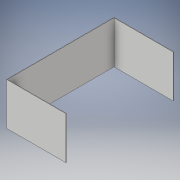
# Autodesk Inventor part: IntakeBackPlate
Saved by Autodesk Inventor 2017 (Build 210142000, 142)
## iProperties
Created: 2020-02-20
Part Number: IntakeBackPlate
Material: Generic
Document SubType Name: Modeling
Designer: S338674153
Density: 1 g/cm^3
Appearance: Default
Author: S338674153
Autodesk Inventor part; units mm, degrees
ref_plane "YZ Plane" through (0, 0, 0) normal (1, 0, 0) x (0, 1, 0)
ref_plane "XZ Plane" through (0, 0, 0) normal (0, 1, 0) x (-1, 0, 0)
ref_plane "XY Plane" through (0, 0, 0) normal (0, 0, 1) x (1, 0, 0)
sketch "Sketch1" plane through (0, 0, 0) normal (0, 1, 0) x (-1, 0, 0)
  line L0 (0, 0) -> (231.775, 0)
  line L1 (231.775, 0) -> (231.775, -4.1774)
  line L2 (229.87, -1.905) -> (0, -1.905)
  line L3 (0, -1.905) -> (0, 0)
  line L4 (231.775, 0) -> (9.6932, 0)
  line L5 (229.87, -1.905) -> (229.87, -417.195)
  line L6 (9.6932, -419.1) -> (231.775, -419.1)
  line L7 (231.775, -419.1) -> (231.775, 0)
  line L8 (231.775, -419.1) -> (0, -419.1)
  line L9 (0, -419.1) -> (0, -417.195)
  line L10 (0, -417.195) -> (229.87, -417.195)
  line L11 (231.775, -13.6272) -> (231.775, -419.1)
  dimension "d0" = 419.1
  dimension "d1" = 231.775
  dimension "d2" = 1.905
  dimension "d3" = 1.905
  dimension "d4" = 1.905
  constraints: 24 end point, 6 parallel, 3 horizontal, 3 perpendicular, 1 point on line
  measures "d0" distance of L6.end L0.end
  measures "d1" distance of L6.end L8.end
  measures "d2" distance of L8.end L9.end
  measures "d3" distance of L2.end L0.start
  measures "d4" distance between parallel lines of L7 L5
extrude "Extrusion1" add sketch "Sketch1" along normal blind 165.1
body "Solid1"
